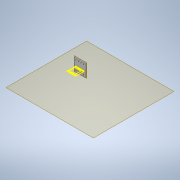
# Autodesk Inventor part: body cover
Saved by Autodesk Inventor 2022 (Build 260153000, 153)
## iProperties
Created: 2022-04-23
Part Number: body cover
Material: Generic
Document SubType Name: Modeling
Designer: efred
Density: 1 g/cm^3
Appearance: Default
Author: efred
Autodesk Inventor part; units mm, degrees
ref_plane "YZ Plane" through (0, 0, 0) normal (1, 0, 0) x (0, 1, 0)
ref_plane "XZ Plane" through (0, 0, 0) normal (0, 1, 0) x (-1, 0, 0)
ref_plane "XY Plane" through (0, 0, 0) normal (0, 0, 1) x (1, 0, 0)
ref_plane "Work Plane1" through (0, 0, 0) normal (0, 0, 1) x (1, 0, 0)
sketch "Sketch1" plane through (0, 0, 0) normal (0, 0, 1) x (1, 0, 0)
  circle A0 centre (-25.75, 18) radius 1.7 projected
  circle A1 centre (4.25, 18) radius 1.7 projected
  circle A2 centre (-15.75, 18) radius 1.7 projected
  circle A3 centre (-5.75, 18) radius 1.7 projected
  line L0 (-32.45, 24.7) -> (12.45, 24.7) construction
  line L1 (-32.45, 13) -> (-32.45, 24.7) construction
  line L2 (-12.45, 13) -> (-32.45, 13) construction
  line L3 (1.25, 8.4548) -> (-12.45, 13) construction
  arc A4 (5.4986, 7.8696) -> (1.25, 8.4548) centre (2.25, 0) ccw construction
  line L4 (12.45, 5) -> (5.4986, 7.8696) construction
  line L5 (12.45, 24.7) -> (12.45, 5) construction
  circle A5 centre (-25.75, -18) radius 1.7 projected
  circle A6 centre (-15.75, -18) radius 1.7 projected
  circle A7 centre (4.25, -18) radius 1.7 projected
  line L6 (12.45, -24.7) -> (-32.45, -24.7) construction
  line L7 (12.45, -5) -> (12.45, -24.7) construction
  line L8 (5.4986, -7.8696) -> (12.45, -5) construction
  arc A8 (1.25, -8.4548) -> (5.4986, -7.8696) centre (2.25, 0) ccw construction
  line L9 (-12.45, -13) -> (1.25, -8.4548) construction
  line L10 (-12.45, -13) -> (-32.45, -13) construction
  line L11 (-32.45, -24.7) -> (-32.45, -13) construction
  circle A9 centre (-5.75, -18) radius 1.7 projected
  line L12 (12.45, 24.7) -> (-32.45, 24.7)
  line L13 (-32.45, 24.7) -> (-32.45, -24.7)
  line L14 (-32.45, -24.7) -> (12.45, -24.7)
  line L15 (12.45, -24.7) -> (12.45, 24.7)
  point P0 (0, 0)
  constraints: 8 end point, 2 parallel, 1 horizontal, 1 perpendicular
extrude "Extrusion1" add sketch "Sketch1" along normal blind 3
ref_plane "Work Plane2" through (-6.9588, 1.65, 41.55) normal (0, 1, 0) x (0, 0, -1)
ref_plane "Work Plane3" through (12.46, 3.65, 25.725) normal (0, 1, 0) x (0, 0, -1)
sketch "Sketch2" plane through (-6.9588, 1.65, 41.55) normal (0, 1, 0) x (0, 0, -1)
  arc A0 (29.75, -19.4088) -> (30.75, -18.4088) centre (29.75, -18.4088) ccw construction
  line L0 (30.75, -18.4088) -> (30.75, -6.9173) construction
  arc A1 (30.75, -6.9173) -> (29.8938, -5.9277) centre (29.75, -6.9173) ccw construction
  arc A2 (29.8938, 0.01) -> (29.8938, -5.9277) centre (30.325, -2.9588) ccw construction
  arc A3 (29.8938, 0.01) -> (30.75, 0.9996) centre (29.75, 0.9996) ccw construction
  line L1 (30.75, 0.9996) -> (30.75, 13.5412) construction
  arc A4 (30.75, 13.5412) -> (29.75, 14.5412) centre (29.75, 13.5412) ccw construction
  line L2 (1.9, 14.5412) -> (29.75, 14.5412) construction
  arc A5 (1.9, 14.5412) -> (0.9, 13.5412) centre (1.9, 13.5412) ccw construction
  line L3 (0.9, 13.5412) -> (0.9, 0.9996) construction
  arc A6 (0.9, 0.9996) -> (1.7563, 0.01) centre (1.9, 0.9996) ccw construction
  arc A7 (1.7563, -5.9277) -> (1.7563, 0.01) centre (1.325, -2.9588) ccw construction
  arc A8 (1.7563, -5.9277) -> (0.9, -6.9173) centre (1.9, -6.9173) ccw construction
  line L4 (0.9, -6.9173) -> (0.9, -18.4088) construction
  arc A9 (0.9, -18.4088) -> (1.9, -19.4088) centre (1.9, -18.4088) ccw construction
  line L5 (29.75, -19.4088) -> (1.9, -19.4088) construction
  line L6 (27.025, -11.9588) -> (27.025, -5.2194) construction
  line L7 (4.625, -11.9588) -> (27.025, -11.9588) construction
  line L8 (4.625, -5.2194) -> (4.625, -11.9588) construction
  arc A10 (4.625, -5.2194) -> (4.625, -0.6983) centre (1.325, -2.9588) ccw construction
  line L9 (4.625, -0.6983) -> (4.625, 11.8412) construction
  line L10 (27.025, 11.8412) -> (4.625, 11.8412) construction
  line L11 (27.025, 11.8412) -> (27.025, -0.6983) construction
  arc A11 (27.025, -0.6983) -> (27.025, -5.2194) centre (30.325, -2.9588) ccw construction
  arc A12 (33.55, -6.9286) -> (32.55, -5.9286) centre (32.55, -6.9286) ccw construction
  line L12 (32.55, -5.9286) -> (30.75, -5.9286) construction
  arc A13 (29.8938, -5.9277) -> (30.75, -5.9286) centre (30.325, -2.9588) ccw construction
  arc A14 (30.75, -6.9173) -> (29.8938, -5.9277) centre (29.75, -6.9173) ccw construction
  line L13 (30.75, -18.4088) -> (30.75, -6.9173) construction
  arc A15 (29.75, -19.4088) -> (30.75, -18.4088) centre (29.75, -18.4088) ccw construction
  line L14 (32.55, -19.4088) -> (29.75, -19.4088) construction
  arc A16 (32.55, -19.4088) -> (33.55, -18.4088) centre (32.55, -18.4088) ccw construction
  line L15 (33.55, -6.9286) -> (33.55, -18.4088) construction
  arc A17 (32.55, 0.0109) -> (33.55, 1.0109) centre (32.55, 1.0109) ccw construction
  line L16 (33.55, 13.5412) -> (33.55, 1.0109) construction
  arc A18 (33.55, 13.5412) -> (32.55, 14.5412) centre (32.55, 13.5412) ccw construction
  line L17 (29.75, 14.5412) -> (32.55, 14.5412) construction
  arc A19 (30.75, 13.5412) -> (29.75, 14.5412) centre (29.75, 13.5412) ccw construction
  line L18 (30.75, 0.9996) -> (30.75, 13.5412) construction
  arc A20 (29.8938, 0.01) -> (30.75, 0.9996) centre (29.75, 0.9996) ccw construction
  arc A21 (30.75, 0.0109) -> (29.8938, 0.01) centre (30.325, -2.9588) ccw construction
  line L19 (30.75, 0.0109) -> (32.55, 0.0109) construction
  arc A22 (-1.9, 1.0109) -> (-0.9, 0.0109) centre (-0.9, 1.0109) ccw construction
  line L20 (-0.9, 0.0109) -> (0.9, 0.0109) construction
  arc A23 (1.7563, 0.01) -> (0.9, 0.0109) centre (1.325, -2.9588) ccw construction
  arc A24 (0.9, 0.9996) -> (1.7563, 0.01) centre (1.9, 0.9996) ccw construction
  line L21 (0.9, 13.5412) -> (0.9, 0.9996) construction
  arc A25 (1.9, 14.5412) -> (0.9, 13.5412) centre (1.9, 13.5412) ccw construction
  line L22 (-0.9, 14.5412) -> (1.9, 14.5412) construction
  arc A26 (-0.9, 14.5412) -> (-1.9, 13.5412) centre (-0.9, 13.5412) ccw construction
  line L23 (-1.9, 1.0109) -> (-1.9, 13.5412) construction
  arc A27 (-0.9, -5.9286) -> (-1.9, -6.9286) centre (-0.9, -6.9286) ccw construction
  line L24 (-1.9, -18.4088) -> (-1.9, -6.9286) construction
  arc A28 (-1.9, -18.4088) -> (-0.9, -19.4088) centre (-0.9, -18.4088) ccw construction
  line L25 (1.9, -19.4088) -> (-0.9, -19.4088) construction
  arc A29 (0.9, -18.4088) -> (1.9, -19.4088) centre (1.9, -18.4088) ccw construction
  line L26 (0.9, -6.9173) -> (0.9, -18.4088) construction
  arc A30 (1.7563, -5.9277) -> (0.9, -6.9173) centre (1.9, -6.9173) ccw construction
  arc A31 (0.9, -5.9286) -> (1.7563, -5.9277) centre (1.325, -2.9588) ccw construction
  line L27 (0.9, -5.9286) -> (-0.9, -5.9286) construction
  line L28 (-1.9, -6.9286) -> (-1.9, 1.0109) construction
  arc A32 (-0.9, -5.9286) -> (-1.9, -6.9286) centre (-0.9, -6.9286) ccw construction
  line L29 (0.9, -5.9286) -> (-0.9, -5.9286) construction
  arc A33 (0.9, -5.9286) -> (0.9, 0.0109) centre (1.325, -2.9588) ccw construction
  line L30 (-0.9, 0.0109) -> (0.9, 0.0109) construction
  arc A34 (-1.9, 1.0109) -> (-0.9, 0.0109) centre (-0.9, 1.0109) ccw construction
  circle A35 centre (1.325, -2.9588) radius 1.725 construction
  line L31 (33.55, 1.0109) -> (33.55, -6.9286) construction
  arc A36 (32.55, 0.0109) -> (33.55, 1.0109) centre (32.55, 1.0109) ccw construction
  line L32 (30.75, 0.0109) -> (32.55, 0.0109) construction
  arc A37 (30.75, 0.0109) -> (30.75, -5.9286) centre (30.325, -2.9588) ccw construction
  line L33 (32.55, -5.9286) -> (30.75, -5.9286) construction
  arc A38 (33.55, -6.9286) -> (32.55, -5.9286) centre (32.55, -6.9286) ccw construction
  circle A39 centre (30.325, -2.9588) radius 1.725 construction
  line L34 (-2.3, 14.5412) -> (0.7, 14.5412)
  line L35 (0.7, -19.4088) -> (-2.3, -19.4088)
  line L36 (-2.3, -19.4088) -> (-2.3, 14.5412)
  line L37 (15.825, 14.5412) -> (15.825, -19.4088) construction
  circle A40 centre (1.325, -2.9588) radius 2.025
  line L38 (0.7, 14.5412) -> (0.7, -1.0327)
  line L39 (0.7, -4.885) -> (0.7, -19.4088)
  arc A41 (30.75, 13.5412) -> (29.75, 14.5412) centre (29.75, 13.5412) ccw construction
  line L40 (30.75, 13.5412) -> (30.75, 0.9996) construction
  arc A42 (29.8938, 0.01) -> (30.75, 0.9996) centre (29.75, 0.9996) ccw construction
  arc A43 (29.8938, 0.01) -> (29.8938, -5.9277) centre (30.325, -2.9588) ccw construction
  arc A44 (30.75, -6.9173) -> (29.8938, -5.9277) centre (29.75, -6.9173) ccw construction
  line L41 (30.75, -6.9173) -> (30.75, -18.4088) construction
  arc A45 (29.75, -19.4088) -> (30.75, -18.4088) centre (29.75, -18.4088) ccw construction
  line L42 (27.025, -5.2194) -> (27.025, -11.9588) construction
  arc A46 (27.025, -0.6983) -> (27.025, -5.2194) centre (30.325, -2.9588) ccw construction
  line L43 (27.025, -0.6983) -> (27.025, 11.8412) construction
  arc A47 (32.55, 0.0109) -> (33.55, 1.0109) centre (32.55, 1.0109) ccw construction
  line L44 (32.55, 0.0109) -> (30.75, 0.0109) construction
  arc A48 (30.75, 0.0109) -> (29.8938, 0.01) centre (30.325, -2.9588) ccw construction
  arc A49 (29.8938, 0.01) -> (30.75, 0.9996) centre (29.75, 0.9996) ccw construction
  line L45 (30.75, 13.5412) -> (30.75, 0.9996) construction
  arc A50 (30.75, 13.5412) -> (29.75, 14.5412) centre (29.75, 13.5412) ccw construction
  line L46 (32.55, 14.5412) -> (29.75, 14.5412) construction
  arc A51 (33.55, 13.5412) -> (32.55, 14.5412) centre (32.55, 13.5412) ccw construction
  line L47 (33.55, 1.0109) -> (33.55, 13.5412) construction
  arc A52 (33.55, -6.9286) -> (32.55, -5.9286) centre (32.55, -6.9286) ccw construction
  line L48 (33.55, -18.4088) -> (33.55, -6.9286) construction
  arc A53 (32.55, -19.4088) -> (33.55, -18.4088) centre (32.55, -18.4088) ccw construction
  line L49 (29.75, -19.4088) -> (32.55, -19.4088) construction
  arc A54 (29.75, -19.4088) -> (30.75, -18.4088) centre (29.75, -18.4088) ccw construction
  line L50 (30.75, -6.9173) -> (30.75, -18.4088) construction
  arc A55 (30.75, -6.9173) -> (29.8938, -5.9277) centre (29.75, -6.9173) ccw construction
  arc A56 (29.8938, -5.9277) -> (30.75, -5.9286) centre (30.325, -2.9588) ccw construction
  line L51 (30.75, -5.9286) -> (32.55, -5.9286) construction
  line L52 (33.55, -6.9286) -> (33.55, 1.0109) construction
  arc A57 (33.55, -6.9286) -> (32.55, -5.9286) centre (32.55, -6.9286) ccw construction
  line L53 (30.75, -5.9286) -> (32.55, -5.9286) construction
  arc A58 (30.75, 0.0109) -> (30.75, -5.9286) centre (30.325, -2.9588) ccw construction
  line L54 (32.55, 0.0109) -> (30.75, 0.0109) construction
  arc A59 (32.55, 0.0109) -> (33.55, 1.0109) centre (32.55, 1.0109) ccw construction
  circle A60 centre (30.325, -2.9588) radius 1.725 construction
  line L55 (33.95, 14.5412) -> (30.95, 14.5412)
  line L56 (30.95, -19.4088) -> (33.95, -19.4088)
  line L57 (33.95, -19.4088) -> (33.95, 14.5412)
  circle A61 centre (30.325, -2.9588) radius 2.025
  line L58 (30.95, 14.5412) -> (30.95, -1.0327)
  line L59 (30.95, -4.885) -> (30.95, -19.4088)
extrude "Extrusion2" add sketch "Sketch2" along normal up to surface (2 mm away) contours L34 L38 A40 L39 L35 L36 | L57 L56 L59 A61 L58 L55
sketch "Sketch3" plane through (-21.5, 3.65, 43.85) normal (0, 1, 0) x (1, 0, 0)
  line L0 (33.95, 0) -> (0, 0) projected
  line L1 (33.95, 36.25) -> (33.95, 33.25) projected
  line L2 (0, 0) -> (33.95, 0)
  line L3 (33.95, 0) -> (33.95, 36.25)
  line L4 (33.95, 36.25) -> (0, 36.25)
  line L5 (0, 36.25) -> (0, 0)
  arc A0 (15.5739, 3) -> (19.4261, 3) centre (17.5, 3.625) ccw projected
  arc A1 (19.4261, 33.25) -> (15.5739, 33.25) centre (17.5, 32.625) ccw projected
  circle A2 centre (17.5, 3.625) radius 2.025
  circle A3 centre (17.5, 32.625) radius 2.025
  circle A4 centre (17.5, 18.125) radius 5
  point P0 (21.5, 43.85)
  point P1 (33.95, 0)
  point P2 (33.95, 33.25)
  point P3 (19.4261, 33.25)
  point P4 (19.4261, 3)
  point P5 (0, 18.125)
  dimension "d15" = 10
  constraints: 8 end point, 2 coincident, 2 parallel, 1 centre point, 1 horizontal, 1 horizontal alignment, 1 midpoint, 1 perpendicular, 1 vertical alignment, 6 other
  measures "d15" diameter of A4
extrude "Extrusion3" add sketch "Sketch3" along normal blind 3
sketch "Sketch4" plane through (12.45, 1.65, 7.6) normal (0, 0, -1) x (-1, 0, 0)
  line L0 (0, 0) -> (0, 5) projected
  line L1 (0, 0) -> (33.95, 0) projected
  line L2 (33.95, 0) -> (33.95, 5) projected
  line L3 (0, 5) -> (33.95, 5) projected
  point P0 (12.45, -1.65)
extrude "Extrusion4" add sketch "Sketch4" along normal up to surface (4.6 mm away)
fillet "Fillet1" radius 4 2 edges at (-4.525, 1.65, 3) (-4.525, 6.65, 3)
body "Solid1"
